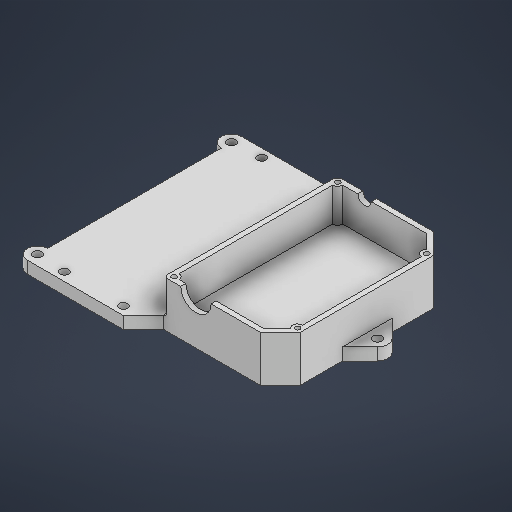
# Autodesk Inventor part: DriverFesting2
Saved by Autodesk Inventor 2026.1 (Build 301233000, 233)
## iProperties
Created: 2026-01-13
Part Number: DriverFesting2
Material: Generic
Document SubType Name: Modeling
Designer: Brynjar
Density: 1 g/cm^3
Appearance: Default
Author: Brynjar
Autodesk Inventor part; units mm, degrees
ref_plane "YZ Plane" through (0, 0, 0) normal (1, 0, 0) x (0, 1, 0)
ref_plane "XZ Plane" through (0, 0, 0) normal (0, 1, 0) x (-1, 0, 0)
ref_plane "XY Plane" through (0, 0, 0) normal (0, 0, 1) x (1, 0, 0)
sketch "Sketch1" plane through (0, 0, 0) normal (0, 1, 0) x (-1, 0, 0)
  line L0 (17.5, 58.5) -> (-17.5, 58.5) construction
  line L1 (-17.5, 58.5) -> (-17.5, -58.5) construction
  line L2 (-17.5, -58.5) -> (17.5, -58.5) construction
  line L3 (17.5, -58.5) -> (17.5, 58.5) construction
  line L4 (17.5, 58.5) -> (-17.5, -58.5) construction
  line L5 (-17.5, 58.5) -> (17.5, -58.5) construction
  circle A0 centre (17.5, -58.5) radius 2.5
  circle A1 centre (-17.5, -58.5) radius 2.5
  circle A2 centre (-17.5, 58.5) radius 2.5
  circle A3 centre (17.5, 58.5) radius 2.5
  line L6 (-34.5, -51.5) -> (34.5, -51.5) construction
  line L7 (34.5, -51.5) -> (34.5, 51.5)
  line L8 (34.5, 51.5) -> (-34.5, 51.5) construction
  line L9 (-34.5, 51.5) -> (-34.5, -51.5) construction
  line L10 (-34.5, -51.5) -> (34.5, 51.5) construction
  line L11 (34.5, -51.5) -> (-34.5, 51.5) construction
  line L12 (22.5, -63.5) -> (-22.5, -63.5)
  line L13 (-22.5, -63.5) -> (-34.5, -51.5)
  line L14 (22.5, -63.5) -> (34.5, -51.5) construction
  line L15 (34.5, 51.5) -> (22.5, 63.5) construction
  line L16 (22.5, 63.5) -> (-22.5, 63.5)
  line L17 (-22.5, 63.5) -> (-34.5, 51.5)
  line L18 (-34.5, -51.5) -> (-91.5, -51.5)
  line L19 (-91.5, 51.5) -> (-34.5, 51.5)
  line L20 (-103.5, -39.5) -> (-103.5, -14.7267)
  line L21 (-91.5, -51.5) -> (-103.5, -39.5)
  line L22 (-103.5, 39.5) -> (-91.5, 51.5)
  circle A4 centre (34.5, -57.5) radius 2.6
  arc A5 (34.5, -63.5) -> (34.5, -51.5) centre (34.5, -57.5) ccw
  line L23 (34.5, -63.5) -> (22.5, -63.5)
  arc A6 (34.5, 51.5) -> (34.5, 63.5) centre (34.5, 57.5) ccw
  line L24 (34.5, 63.5) -> (22.5, 63.5)
  circle A7 centre (34.5, 57.5) radius 2.6
  circle A8 centre (-109.6, 0) radius 2.6
  line L25 (-103.5, -14.7267) -> (-113.9134, -4.3134)
  line L26 (-103.5, 14.7267) -> (-113.9134, 4.3134)
  arc A9 (-113.9134, 4.3134) -> (-113.9134, -4.3134) centre (-109.6, 0) ccw
  line L27 (-107, 0) -> (-103.5, 0) construction
  line L28 (-112.2, 0) -> (-115.7, 0) construction
  line L29 (-103.5, -14.7267) -> (-103.5, 14.7267) construction
  line L30 (-103.5, 14.7267) -> (-103.5, 39.5)
  point P0 (0, 0)
  point P1 (-103.5, -51.5)
  point P2 (-103.5, 51.5)
  dimension "d0" = 35
  dimension "d1" = 117
  dimension "d2" = 5
  dimension "d3" = 69
  dimension "d4" = 103
  dimension "d5" = 5
  dimension "d10" = 12
  dimension "d12" = 69
  dimension "d13" = 5.2
  dimension "d15" = 3.5
  constraints: 62 end point, 10 centre point, 9 point on circle, 8 perpendicular, 8 point on line, 7 coincident, 6 parallel, 6 tangent, 5 equal length, 5 equal radius, 5 midpoint, 4 horizontal, 3 vertical, 2 collinear
  measures "d0" distance of L2.end L1.end
  measures "d1" distance of L1.end L0.end
  measures "d2" diameter of A3
  measures "d3" distance of L7.end L8.end
  measures "d4" distance of L6.end L7.end
  measures "d5" distance from line of L16 L0.start
  measures "d10" distance of point (-103.5, -51.5) L18.end
  measures "d12" distance between parallel lines of L20 L9
  measures "d13" diameter of A4
  measures "d15" distance of L28.start L28.end
extrude "Extrusion1" add sketch "Sketch1" against normal blind 6.2
sketch "Sketch2" plane through (0, 0, 0) normal (0, 1, 0) x (1, 0, 0)
  circle A0 centre (-17.5, -58.5) radius 2.5 construction
  circle A1 centre (17.5, -58.5) radius 2.5 construction
  circle A2 centre (-17.5, 58.5) radius 2.5 construction
  circle A3 centre (17.5, 58.5) radius 2.5 construction
  circle A4 centre (-17.5, -58.5) radius 4.25
  circle A5 centre (-17.5, 58.5) radius 4.25
  circle A6 centre (17.5, 58.5) radius 4.25
  circle A7 centre (17.5, -58.5) radius 4.25
  point P0 (0, 0)
  dimension "d18" = 8.5
  constraints: 4 centre point, 4 coincident, 3 equal radius
  measures "d18" diameter of A4
extrude "Extrusion2" [suppressed]
sketch "Sketch3" plane through (0, -6.2, 0) normal (0, -1, 0) x (1, 0, 0)
  line L0 (-34.5, 51.5) -> (-34.5, -51.5) projected
  arc A0 (-34.5, -51.5) -> (-34.5, -63.5) centre (-34.5, -57.5) ccw projected
  line L1 (-34.5, -63.5) -> (22.5, -63.5) projected
  line L2 (22.5, -63.5) -> (34.5, -51.5) projected
  line L3 (34.5, -51.5) -> (91.5, -51.5) projected
  line L4 (91.5, -51.5) -> (103.5, -39.5) projected
  line L5 (103.5, -39.5) -> (103.5, -14.7267) projected
  line L6 (103.5, -14.7267) -> (113.9134, -4.3134) projected
  arc A1 (113.9134, -4.3134) -> (113.9134, 4.3134) centre (109.6, 0) ccw projected
  line L7 (113.9134, 4.3134) -> (103.5, 14.7267) projected
  line L8 (103.5, 14.7267) -> (103.5, 39.5) projected
  line L9 (103.5, 39.5) -> (91.5, 51.5) projected
  line L10 (91.5, 51.5) -> (34.5, 51.5) projected
  line L11 (34.5, 51.5) -> (22.5, 63.5) projected
  line L12 (22.5, 63.5) -> (-34.5, 63.5) projected
  arc A2 (-34.5, 63.5) -> (-34.5, 51.5) centre (-34.5, 57.5) ccw projected
  circle A3 centre (-17.5, -58.5) radius 2.5 construction
  circle A4 centre (17.5, -58.5) radius 2.5 construction
  circle A5 centre (17.5, 58.5) radius 2.5 construction
  circle A6 centre (-17.5, 58.5) radius 2.5 construction
  circle A7 centre (109.6, 0) radius 2.6 projected
  circle A8 centre (-34.5, 57.5) radius 2.6 projected
  circle A9 centre (-34.5, -57.5) radius 2.6 projected
  point P0 (0, 0)
extrude "Extrusion3" add sketch "Sketch3" along normal blind 1
sketch "Sketch4" plane through (0, 0, 0) normal (0, 1, 0) x (1, 0, 0)
  line L0 (34.5, -51.5) -> (34.5, 51.5) projected
  line L1 (34.5, 51.5) -> (91.5, 51.5) projected
  line L2 (103.5, 39.5) -> (91.5, 51.5) projected
  line L3 (103.5, 14.7267) -> (103.5, 39.5) projected
  line L4 (103.5, 14.7267) -> (103.5, -14.7267) projected
  line L5 (103.5, -39.5) -> (103.5, -14.7267) projected
  line L6 (91.5, -51.5) -> (103.5, -39.5) projected
  line L7 (34.5, -51.5) -> (91.5, -51.5) projected
  circle A0 centre (37.5, 48.5) radius 1.5
  circle A1 centre (100.5, 38.2574) radius 1.5
  circle A2 centre (100.5, -38.2574) radius 1.5
  circle A3 centre (37.5, -48.5) radius 1.5
  arc A4 (40.5, 48.5) -> (37.5, 45.5) centre (37.5, 48.5) ccw construction
  arc A5 (100.5, 35.2574) -> (98.3787, 40.3787) centre (100.5, 38.2574) ccw construction
  arc A6 (98.3787, -40.3787) -> (100.5, -35.2574) centre (100.5, -38.2574) ccw construction
  arc A7 (37.5, -45.5) -> (40.5, -48.5) centre (37.5, -48.5) ccw construction
  line L8 (40.5, 48.5) -> (90.2574, 48.5)
  line L9 (37.5, 45.5) -> (37.5, -45.5)
  line L10 (40.5, -48.5) -> (90.2574, -48.5)
  line L11 (90.2574, -48.5) -> (98.3787, -40.3787)
  line L12 (100.5, -35.2574) -> (100.5, 35.2574)
  line L13 (98.3787, 40.3787) -> (90.2574, 48.5)
  arc A8 (37.5, 45.5) -> (40.5, 48.5) centre (37.5, 48.5) ccw
  arc A9 (98.3787, 40.3787) -> (100.5, 35.2574) centre (100.5, 38.2574) ccw
  arc A10 (100.5, -35.2574) -> (98.3787, -40.3787) centre (100.5, -38.2574) ccw
  arc A11 (40.5, -48.5) -> (37.5, -45.5) centre (37.5, -48.5) ccw
  line L14 (34.5, -49.7426) -> (36.2574, -51.5)
  line L15 (34.5, 49.7426) -> (36.2574, 51.5)
  point P0 (0, 0)
  dimension "d24" = 3
  dimension "d25" = 3
  constraints: 16 end point, 16 point on circle, 12 centre point, 12 point on line, 10 tangent, 6 equal radius, 4 coincident, 2 horizontal, 2 parallel, 2 perpendicular
  measures "d24" diameter of A0
  measures "d25" distance between parallel lines of L1 L8
extrude "Extrusion4" add sketch "Sketch4" along normal blind 20 contours L0 L15 L1 L2 L3 L4 L5 L6 L7 L14
sketch "Sketch7" plane through (0, 20, 0) normal (0, 1, 0) x (1, 0, 0)
  line L0 (91.5, 51.5) -> (36.2574, 51.5) projected
  line L1 (36.2574, 51.5) -> (34.5, 49.7426) projected
  line L2 (34.5, 49.7426) -> (34.5, -49.7426) projected
  line L3 (34.5, -49.7426) -> (36.2574, -51.5) projected
  line L4 (36.2574, -51.5) -> (91.5, -51.5) projected
  line L5 (91.5, -51.5) -> (103.5, -39.5) projected
  line L6 (103.5, -39.5) -> (103.5, 39.5) projected
  line L7 (103.5, 39.5) -> (91.5, 51.5) projected
  arc A0 (37.5, 45.5) -> (40.5, 48.5) centre (37.5, 48.5) ccw projected
  line L8 (40.5, 48.5) -> (90.2574, 48.5) projected
  line L9 (90.2574, 48.5) -> (98.3787, 40.3787) projected
  arc A1 (98.3787, 40.3787) -> (100.5, 35.2574) centre (100.5, 38.2574) ccw projected
  line L10 (100.5, 35.2574) -> (100.5, -35.2574) projected
  arc A2 (100.5, -35.2574) -> (98.3787, -40.3787) centre (100.5, -38.2574) ccw projected
  line L11 (98.3787, -40.3787) -> (90.2574, -48.5) projected
  line L12 (90.2574, -48.5) -> (40.5, -48.5) projected
  arc A3 (40.5, -48.5) -> (37.5, -45.5) centre (37.5, -48.5) ccw projected
  line L13 (37.5, -45.5) -> (37.5, 45.5) projected
  circle A4 centre (37.5, -48.5) radius 1.5 construction
  circle A5 centre (100.5, -38.2574) radius 1.5 construction
  circle A6 centre (100.5, 38.2574) radius 1.5 construction
  circle A7 centre (37.5, 48.5) radius 1.5 construction
  circle A8 centre (37.5, 48.5) radius 1.7
  circle A9 centre (100.5, 38.2574) radius 1.7
  circle A10 centre (100.5, -38.2574) radius 1.7
  circle A11 centre (37.5, -48.5) radius 1.7
  point P0 (0, 0)
  dimension "d35" = 0.2
  constraints: 4 centre point, 4 coincident, 3 equal radius
  measures "d35" radial gap between concentric circles of A8 A7
extrude "Extrusion5" add sketch "Sketch7" along normal blind 17 separate body
sketch "Sketch8" plane through (0, 37, 0) normal (0, 1, 0) x (1, 0, 0)
  line L0 (36.2574, 51.5) -> (34.5, 49.7426) projected
  line L1 (34.5, 49.7426) -> (34.5, -49.7426) projected
  line L2 (34.5, -49.7426) -> (36.2574, -51.5) projected
  line L3 (36.2574, -51.5) -> (91.5, -51.5) projected
  line L4 (91.5, -51.5) -> (103.5, -39.5) projected
  line L5 (103.5, -39.5) -> (103.5, 39.5) projected
  line L6 (103.5, 39.5) -> (91.5, 51.5) projected
  line L7 (91.5, 51.5) -> (36.2574, 51.5) projected
  circle A0 centre (37.5, -48.5) radius 1.7 projected
  circle A1 centre (100.5, -38.2574) radius 1.7 projected
  circle A2 centre (100.5, 38.2574) radius 1.7 projected
  circle A3 centre (37.5, 48.5) radius 1.7 projected
  arc A4 (37.5, 45.5) -> (40.5, 48.5) centre (37.5, 48.5) ccw construction
  line L8 (40.5, 48.5) -> (90.2574, 48.5) construction
  line L9 (90.2574, 48.5) -> (98.3787, 40.3787) construction
  arc A5 (98.3787, 40.3787) -> (100.5, 35.2574) centre (100.5, 38.2574) ccw construction
  line L10 (100.5, 35.2574) -> (100.5, -35.2574) construction
  arc A6 (100.5, -35.2574) -> (98.3787, -40.3787) centre (100.5, -38.2574) ccw construction
  line L11 (98.3787, -40.3787) -> (90.2574, -48.5) construction
  line L12 (90.2574, -48.5) -> (40.5, -48.5) construction
  arc A7 (40.5, -48.5) -> (37.5, -45.5) centre (37.5, -48.5) ccw construction
  line L13 (37.5, -45.5) -> (37.5, 45.5) construction
  point P0 (0, 0)
extrude "Extrusion6" add sketch "Sketch8" along normal blind 2 bodies 2
chamfer "Chamfer1" distance 1.2426 angle 45 2 edges at (35.3787, 0, 50.6213) (35.3787, 0, -50.6213)
sketch "Sketch6" plane through (34.5, -7.2, 51.5) normal (0, 0, 1) x (1, 0, 0)
  circle A0 centre (19, 27.2) radius 9
  line L0 (0, 8.4426) -> (0, 27.2) construction
  line L1 (10, 27.2) -> (0, 27.2) construction
  line L2 (6, 7.2) -> (55.7574, 7.2) construction
  line L3 (19, 7.2) -> (19, 18.2) construction
  point P0 (-34.5, 7.2)
  dimension "d31" = 18
  dimension "d32" = 10
  dimension "d34" = 20
  constraints: 4 end point, 4 point on line, 2 point on circle, 1 centre point, 1 perpendicular, 1 vertical
  measures "d31" diameter of A0
  measures "d32" distance of L1.start L1.end
  measures "d34" distance between parallel lines of L2 L1
extrude "Extrusion7" cut sketch "Sketch6" against normal up to surface (3 mm away) bodies 1 2
sketch "Sketch9" plane through (91.5, -7.2, -51.5) normal (0, 0, -1) x (-1, 0, 0)
  arc A0 (29, 27.2) -> (47, 27.2) centre (38, 27.2) ccw construction
  circle A1 centre (38, 27.2) radius 4
  point P0 (91.5, 7.2)
  dimension "d42" = 8
  constraints: 1 centre point, 1 coincident
  measures "d42" diameter of A1
extrude "Extrusion8" cut sketch "Sketch9" against normal up to surface (3 mm away) bodies 1 2
body "Solid1"
body "Solid2"
